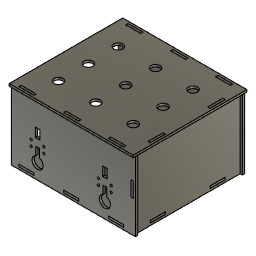
Chasis 4 with motor slots (Autodesk Fusion 360 design; units mm, degrees)
Autodesk Fusion 360 part; units mm, degrees
sketch "Sketch1" plane through (0, 0, 0) normal (0, 0, 1) x (1, 0, 0)
  line L0 (0, 0) -> (160, 0)
  line L1 (160, 0) -> (160, 140)
  line L2 (160, 140) -> (0, 140)
  line L3 (0, 140) -> (0, 0)
  line L4 (70, 0) -> (90, 0)
  line L5 (90, 0) -> (90, -3)
  line L6 (90, -3) -> (70, -3)
  line L7 (70, -3) -> (70, 0)
  line L8 (80, 0) -> (80, 24.5261)
  line L9 (0, 70) -> (20, 70)
  line L10 (150, -3) -> (130, -3)
  line L11 (130, -3) -> (130, 0)
  line L12 (150, 0) -> (150, -3)
  line L13 (30, -3) -> (10, -3)
  line L14 (10, -3) -> (10, 0)
  line L15 (30, 0) -> (30, -3)
  line L16 (0, 50) -> (0, 70)
  line L17 (10, 143) -> (10, 140)
  line L18 (30, 143) -> (10, 143)
  line L19 (30, 140) -> (30, 143)
  line L20 (70, 143) -> (70, 140)
  line L21 (90, 143) -> (70, 143)
  line L22 (90, 140) -> (90, 143)
  line L23 (130, 143) -> (130, 140)
  line L24 (150, 143) -> (130, 143)
  line L25 (150, 140) -> (150, 143)
  line L26 (160, 120) -> (163, 120)
  line L27 (163, 120) -> (163, 100)
  line L28 (163, 100) -> (160, 100)
  line L29 (160, 40) -> (163, 40)
  line L30 (163, 40) -> (163, 20)
  line L31 (163, 20) -> (160, 20)
  dimension "d1" = 140
  dimension "d2" = 3
  dimension "d3" = 20
  dimension "d6" = 0
  dimension "d7" = 60
  dimension "d71" = 140
  dimension "d72" = 140
  constraint horizontal L0
  constraint vertical L1
  constraint horizontal L2
  constraint vertical L3
  constraint coincident L0.start L3.end
  constraint horizontal L4
  constraint vertical L5
  constraint horizontal L6
  constraint vertical L7
  constraint coincident L0 L4.start
  constraint midpoint L0 L8.start
  constraint perpendicular L4 L8
  constraint midpoint L3 L9.start
  constraint perpendicular L3 L9
  constraint vertical L16
  constraint coincident L3 L9.start
  constraint symmetric L4.start L9 L20.end
  constraint symmetric L4.end L9 L22.start
  constraint symmetric L5.end L9 L21.start
  constraint symmetric L6.end L9 L20.start
  constraint symmetric L9 L10.start L24.start
  constraint symmetric L9 L10.end L23.start
  constraint symmetric L9 L11.end L23.end
  constraint symmetric L9 L12.start L25.start
  constraint symmetric L9 L13.start L18.start
  constraint symmetric L9 L13.end L17.start
  constraint symmetric L9 L14.end L17.end
  constraint symmetric L9 L15.start L19.start
  measures "d1" distance of L0.end L1.end
  measures "d2" distance of L4.end L5.end
  measures "d3" distance of L5.end L6.end
  measures "d71" distance of L0.end L1.end
  measures "d72" distance of L0.end L1.end
extrude "Extrude1" add sketch "Sketch1" along normal blind 3 makes body 1
sketch "Sketch2" plane through (0, 0, 0) normal (0, -1, 0) x (1, 0, 0)
  line L0 (0, 0) -> (10, 0)
  line L1 (10, 0) -> (10, 3)
  line L2 (10, 3) -> (0, 3)
  line L3 (0, 3) -> (0, 0)
  line L4 (0, -5) -> (168, -5)
  line L5 (168, -5) -> (168, 90)
  line L6 (168, 90) -> (0, 90)
  line L7 (0, 90) -> (0, -5)
  line L8 (70, 90) -> (90, 90)
  line L9 (90, 90) -> (90, 93)
  line L10 (90, 93) -> (70, 93)
  line L11 (70, 93) -> (70, 90)
  line L12 (30, 93) -> (10, 93)
  line L13 (10, 93) -> (10, 90)
  line L14 (30, 90) -> (30, 93)
  line L15 (150, 93) -> (130, 93)
  line L16 (130, 93) -> (130, 90)
  line L17 (150, 90) -> (150, 93)
  line L18 (0, -5) -> (168, -5)
  line L19 (168, -5) -> (168, -3)
  line L20 (168, -3) -> (0, -3)
  line L21 (0, -3) -> (0, -5)
  dimension "d15" = 168
  dimension "d16" = 95
  dimension "d17" = 20
  dimension "d18" = 3
  dimension "d21" = 60
  dimension "d22" = 0
  dimension "d85" = 2
  constraint horizontal L4
  constraint vertical L5
  constraint horizontal L6
  constraint vertical L7
  constraint horizontal L8
  constraint vertical L9
  constraint horizontal L10
  constraint vertical L11
  constraint coincident L6 L8.start
  constraint horizontal L18
  constraint vertical L19
  constraint horizontal L20
  constraint vertical L21
  measures "d15" distance of L4.start L4.end
  measures "d16" distance of L4.end L5.end
  measures "d17" distance of L9.end L10.end
  measures "d18" distance of L8.end L9.end
  measures "d85" distance of L4.start L20.end
extrude "Extrude2" add sketch "Sketch2" along normal blind 3 separate body makes body 2
sketch "Sketch3" plane through (160, 0, 0) normal (1, 0, 0) x (0, 1, 0)
  line L0 (0, 0) -> (20, 0)
  line L1 (20, 0) -> (20, 3)
  line L2 (20, 3) -> (0, 3)
  line L3 (0, 3) -> (0, 0)
  line L4 (0, -5) -> (140, -5)
  line L5 (140, -5) -> (140, 90)
  line L6 (140, 90) -> (0, 90)
  line L7 (0, 90) -> (0, -5)
  line L8 (20, 90) -> (40, 90)
  line L9 (40, 90) -> (40, 93)
  line L10 (40, 93) -> (20, 93)
  line L11 (20, 93) -> (20, 90)
  line L12 (100, 90) -> (120, 90)
  line L13 (120, 90) -> (120, 93)
  line L14 (120, 93) -> (100, 93)
  line L15 (100, 93) -> (100, 90)
  line L16 (0, 40) -> (-3, 40)
  line L17 (-3, 40) -> (-3, 60)
  line L18 (-3, 60) -> (0, 60)
  line L19 (0, 60) -> (0, 40)
  line L20 (140, 40) -> (143, 40)
  line L21 (143, 40) -> (143, 60)
  line L22 (143, 60) -> (140, 60)
  line L23 (140, 60) -> (140, 40)
  dimension "d33" = 20
  dimension "d34" = 3
  dimension "d35" = 3
  dimension "d36" = 3
  dimension "d37" = 20
  dimension "d38" = 3
  dimension "d74" = 140
  constraint horizontal L4
  constraint vertical L5
  constraint horizontal L6
  constraint vertical L7
  constraint horizontal L8
  constraint vertical L9
  constraint horizontal L10
  constraint vertical L11
  constraint coincident L6 L8.start
  constraint horizontal L12
  constraint vertical L13
  constraint horizontal L14
  constraint vertical L15
  constraint coincident L6 L12.start
  constraint horizontal L16
  constraint vertical L17
  constraint horizontal L18
  constraint vertical L19
  constraint coincident L7 L16.start
  constraint horizontal L20
  constraint vertical L21
  constraint horizontal L22
  constraint vertical L23
  constraint coincident L5 L20.start
  measures "d33" distance of L8.start L8.end
  measures "d34" distance of L8.start L10.end
  measures "d35" distance of L12.start L14.end
  measures "d36" distance of L16.start L16.end
  measures "d37" distance of L16.start L18.end
  measures "d38" distance of L20.start L20.end
  measures "d74" distance of L5 L7
extrude "Extrude5" add sketch "Sketch3" along normal blind 3 separate body contours L5 L20 L21 L22 L23 makes body 3
extrude "Extrude3" add sketch "Sketch3" along normal blind 3 separate body contours L0 L1 L2 L3 L7 | L0 L1 L2 L4 L5 L6 L7 L8 L12 L19 L23 | L7 L16 L17 L18 L19 | L6 L8 L9 L10 L11 | L6 L12 L13 L14 L15 makes body 4
sketch "Sketch5" plane through (0, 140, 0) normal (0, 1, 0) x (-1, 0, 0)
  line L0 (-160, 0) -> (-150, 0)
  line L1 (-150, 0) -> (-150, 3)
  line L2 (-150, 3) -> (-160, 3)
  line L3 (-160, 3) -> (-160, 0)
  line L4 (-168, -5) -> (0, -5)
  line L5 (0, -5) -> (0, 90)
  line L6 (0, 90) -> (-168, 90)
  line L7 (-168, 90) -> (-168, -5)
  line L8 (-150, 90) -> (-130, 90)
  line L9 (-130, 90) -> (-130, 93)
  line L10 (-130, 93) -> (-150, 93)
  line L11 (-150, 93) -> (-150, 90)
  line L12 (-90, 90) -> (-70, 90)
  line L13 (-70, 90) -> (-70, 78)
  line L14 (-70, 78) -> (-90, 78)
  line L15 (-90, 78) -> (-90, 90)
  line L16 (-30, 90) -> (-10, 90)
  line L17 (-10, 90) -> (-10, 78)
  line L18 (-10, 78) -> (-30, 78)
  line L19 (-30, 78) -> (-30, 90)
  dimension "d41" = 20
  dimension "d42" = 3
  constraint horizontal L4
  constraint vertical L5
  constraint horizontal L6
  constraint vertical L7
  constraint horizontal L8
  constraint vertical L9
  constraint horizontal L10
  constraint vertical L11
  constraint coincident L6 L8.start
  constraint horizontal L12
  constraint vertical L13
  constraint horizontal L14
  constraint vertical L15
  constraint coincident L6 L12.start
  constraint horizontal L16
  constraint vertical L17
  constraint horizontal L18
  constraint vertical L19
  constraint coincident L6 L16.start
  measures "d41" distance of L8.start L8.end
  measures "d42" distance of L8.start L10.end
combine "Combine1" operation add target body 4 tool bodies 3
combine "Combine2" [no effect]
sketch "Sketch7" plane through (0, 0, 90) normal (0, 0, 1) x (-1, 0, 0)
  line L0 (-10, 0) -> (0, 0)
  line L1 (0, 0) -> (0, 3)
  line L2 (0, 3) -> (-10, 3)
  line L3 (-10, 3) -> (-10, 0)
  line L4 (0, -128) -> (-168, -128)
  line L5 (-168, -128) -> (-168, 28)
  line L6 (-168, 28) -> (0, 28)
  line L7 (0, 28) -> (0, -128)
  dimension "d73" = 156
  constraint horizontal L4
  constraint vertical L5
  constraint horizontal L6
  constraint vertical L7
  measures "d73" distance of L4.start L6.end
extrude "Extrude8" add sketch "Sketch7" along normal blind 3 separate body makes body 5
combine "Combine4" operation cut target body 2 tool bodies 1 keep tools
combine "Combine5" operation cut target body 4 tool bodies 1 keep tools
combine "Combine6" operation cut target body 5 tool bodies 1 keep tools
combine "Combine7" operation cut target body 5 tool bodies 2 keep tools
combine "Combine8" operation cut target body 5 tool bodies 4 keep tools
combine "Combine9" operation cut target body 2 tool bodies 4 keep tools
sketch "Sketch8" plane through (0, -3, 0) normal (0, -1, 0) x (1, 0, 0)
  line L0 (160, 40) -> (160, 60)
  line L1 (160, 60) -> (163, 60)
  line L2 (163, 60) -> (163, 40)
  line L3 (163, 40) -> (160, 40)
  line L4 (130, 0) -> (130, 3)
  line L5 (130, 3) -> (150, 3)
  line L6 (150, 3) -> (150, 0)
  line L7 (150, 0) -> (130, 0)
  line L8 (70, 0) -> (70, 3)
  line L9 (70, 3) -> (90, 3)
  line L10 (90, 3) -> (90, 0)
  line L11 (90, 0) -> (70, 0)
  line L12 (10, 0) -> (10, 3)
  line L13 (10, 3) -> (30, 3)
  line L14 (30, 3) -> (30, 0)
  line L15 (30, 0) -> (10, 0)
  line L16 (150, 90) -> (150, 93)
  line L17 (150, 93) -> (130, 93)
  line L18 (130, 93) -> (130, 90)
  line L19 (130, 90) -> (90, 90)
  line L20 (90, 90) -> (90, 93)
  line L21 (90, 93) -> (70, 93)
  line L22 (70, 93) -> (70, 90)
  line L23 (70, 90) -> (30, 90)
  line L24 (30, 90) -> (30, 93)
  line L25 (30, 93) -> (10, 93)
  line L26 (10, 93) -> (10, 90)
  line L27 (10, 90) -> (0, 90)
  line L28 (0, 90) -> (0, -5)
  line L29 (0, -5) -> (168, -5)
  line L30 (168, -5) -> (168, 90)
  line L31 (168, 90) -> (150, 90)
  circle A0 centre (35, 17) radius 7.5
  circle A1 centre (125, 17) radius 7.5
  dimension "d54" = 15
  dimension "d55" = 15
  measures "d54" diameter of A1
  measures "d55" diameter of A0
sketch "Sketch9" plane through (0, 0, 93) normal (0, 0, 1) x (-1, 0, 0)
  line L0 (-10, 0) -> (-30, 0)
  line L1 (-30, 0) -> (-30, 3)
  line L2 (-30, 3) -> (-10, 3)
  line L3 (-10, 3) -> (-10, 0)
  line L4 (-70, 0) -> (-90, 0)
  line L5 (-90, 0) -> (-90, 3)
  line L6 (-90, 3) -> (-70, 3)
  line L7 (-70, 3) -> (-70, 0)
  line L8 (-130, 0) -> (-150, 0)
  line L9 (-150, 0) -> (-150, 3)
  line L10 (-150, 3) -> (-130, 3)
  line L11 (-130, 3) -> (-130, 0)
  line L12 (0, 28) -> (-168, 28)
  line L13 (-168, 28) -> (-168, -128)
  line L14 (-168, -128) -> (0, -128)
  line L15 (0, -128) -> (0, 28)
  circle A0 centre (-30, -90) radius 6
  circle A1 centre (-80, -90) radius 6
  circle A2 centre (-130, -90) radius 6
  circle A3 centre (-30, -50) radius 6
  circle A4 centre (-80, -50) radius 6
  circle A5 centre (-130, -50) radius 6
  circle A6 centre (-30, -10) radius 6
  circle A7 centre (-80, -10) radius 6
  circle A8 centre (-130, -10) radius 6
  line L16 (-160, -20) -> (-160, -40)
  line L17 (-160, -40) -> (-163, -40)
  line L18 (-163, -40) -> (-163, -20)
  line L19 (-163, -20) -> (-160, -20)
  line L20 (-160, -100) -> (-160, -120)
  line L21 (-160, -120) -> (-163, -120)
  line L22 (-163, -120) -> (-163, -100)
  line L23 (-163, -100) -> (-160, -100)
  dimension "d58" = 12
  dimension "d61" = -100
  dimension "d62" = 0
  dimension "d65" = 0
  dimension "d66" = 80
  measures "d58" diameter of A0
extrude "Extrude10" cut sketch "Sketch9" against normal blind 3 contours A0 | A1 | A2 | A3 | A4 | A5 | A6 | A7 | A8 bodies 5
extrude "Extrude11" cut sketch "Sketch9" against normal blind 86 contours A1 | A5 | A7 bodies 1
copy_body "CopyPasteBodies1" bodies 2 makes body 6
move_body "Move1" bodies 6 to x (1, 0, 0) y (0, 1, 0) z (0, 0, 1) at (0, 120, 0)
move_body "Move2" bodies 6 to x (1, 0, 0) y (0, 1, 0) z (0, 0, 1) at (0, 3, 0)
move_body "Move3" bodies 5 to x (1, 0, 0) y (0, 1, 0) z (0, 0, 1) at (0, 0, 10)
move_body "Move4" bodies 6 to x (1, 0, 0) y (0, 1, 0) z (0, 0, 1) at (0, 10, 0)
move_body "Move5" bodies 2 to x (1, 0, 0) y (0, 1, 0) z (0, 0, 1) at (0, -10, 0)
move_body "Move6" bodies 4 to x (1, 0, 0) y (0, 1, 0) z (0, 0, 1) at (10, 0, 0)
move_body "Move7" bodies 6 to x (1, 0, 0) y (0, 1, 0) z (0, 0, 1) at (0, 10, 0)
move_body "Move8" bodies 2 to x (1, 0, 0) y (0, 1, 0) z (0, 0, 1) at (0, 10, 0)
move_body "Move9" bodies 5 to x (1, 0, 0) y (0, 1, 0) z (0, 0, 1) at (0, 20, -10)
move_body "Move10" bodies 5 to x (1, 0, 0) y (0, 1, 0) z (0, 0, 1) at (0, 0, 10)
extrude "Extrude12" add 1 faces at (10, 19, 102) along direction (1, 0, 0) blind 20 on bodies 5 bodies 5
extrude "Extrude13" add 1 faces at (70, 19, 102) along direction (1, 0, 0) blind 20 on bodies 5 bodies 5
extrude "Extrude14" add 1 faces at (130, 19, 102) along direction (1, 0, 0) blind 20 on bodies 5 bodies 5
extrude "Extrude15" add 1 faces at (161, 140, 101) along direction (0, -1, 0) blind 20 on bodies 5 bodies 5
extrude "Extrude16" add 1 faces at (161, 60, 101) along direction (0, -1, 0) blind 20 on bodies 5 bodies 5
move_body "Move11" bodies 4 to x (1, 0, 0) y (0, 1, 0) z (0, 0, 1) at (-10, 0, 0)
move_body "Move12" bodies 5 to x (1, 0, 0) y (0, 1, 0) z (0, 0, 1) at (0, 0, -10)
move_body "Move13" bodies 5 to x (1, 0, 0) y (0, 1, 0) z (0, 0, 1) at (0, 0, 10)
move_body "Move14" bodies 5 to x (1, 0, 0) y (0, 1, 0) z (0, 0, 1) at (0, 0, -10)
combine "Combine11" operation cut target body 5 tool bodies 6 keep tools
combine "Combine12" operation cut target body 5 tool bodies 4 keep tools
combine "Combine13" operation cut target body 5 tool bodies 2 keep tools
sketch "Sketch10" plane through (0, -3, 0) normal (0, -1, 0) x (1, 0, 0)
  line L0 (160, 40) -> (160, 60)
  line L1 (160, 60) -> (163, 60)
  line L2 (163, 60) -> (163, 40)
  line L3 (163, 40) -> (160, 40)
  line L4 (130, 0) -> (130, 3)
  line L5 (130, 3) -> (150, 3)
  line L6 (150, 3) -> (150, 0)
  line L7 (150, 0) -> (130, 0)
  line L8 (70, 0) -> (70, 3)
  line L9 (70, 3) -> (90, 3)
  line L10 (90, 3) -> (90, 0)
  line L11 (90, 0) -> (70, 0)
  line L12 (10, 0) -> (10, 3)
  line L13 (10, 3) -> (30, 3)
  line L14 (30, 3) -> (30, 0)
  line L15 (30, 0) -> (10, 0)
  line L16 (150, 90) -> (150, 93)
  line L17 (150, 93) -> (130, 93)
  line L18 (130, 93) -> (130, 90)
  line L19 (130, 90) -> (90, 90)
  line L20 (90, 90) -> (90, 93)
  line L21 (90, 93) -> (70, 93)
  line L22 (70, 93) -> (70, 90)
  line L23 (70, 90) -> (30, 90)
  line L24 (30, 90) -> (30, 93)
  line L25 (30, 93) -> (10, 93)
  line L26 (10, 93) -> (10, 90)
  line L27 (10, 90) -> (0, 90)
  line L28 (0, 90) -> (0, -5)
  line L29 (0, -5) -> (168, -5)
  line L30 (168, -5) -> (168, 90)
  line L31 (168, 90) -> (150, 90)
  line L32 (0, -5) -> (168, -5)
  line L33 (168, -5) -> (168, -3)
  line L34 (168, -3) -> (0, -3)
  line L35 (0, -3) -> (0, -5)
  dimension "d86" = 2
  constraint horizontal L32
  constraint vertical L33
  constraint horizontal L34
  constraint vertical L35
  constraint coincident L28.end L29.start
  measures "d86" distance of L28.end L34.end
extrude "Extrude17" cut sketch "Sketch10" against normal blind 146 contours L28 L29 L30 L32 L33 L34 L35 bodies 2 4 6
sketch "Sketch11" plane through (0, -3, 0) normal (0, -1, 0) x (1, 0, 0)
  line L0 (0, -3) -> (168, -3)
  line L1 (168, -3) -> (168, 90)
  line L2 (168, 90) -> (150, 90)
  line L3 (150, 90) -> (150, 93)
  line L4 (150, 93) -> (130, 93)
  line L5 (130, 93) -> (130, 90)
  line L6 (130, 90) -> (90, 90)
  line L7 (90, 90) -> (90, 93)
  line L8 (90, 93) -> (70, 93)
  line L9 (70, 93) -> (70, 90)
  line L10 (70, 90) -> (30, 90)
  line L11 (30, 90) -> (30, 93)
  line L12 (30, 93) -> (10, 93)
  line L13 (10, 93) -> (10, 90)
  line L14 (10, 90) -> (0, 90)
  line L15 (0, 90) -> (0, -3)
  line L16 (160, 40) -> (160, 60)
  line L17 (160, 60) -> (163, 60)
  line L18 (163, 60) -> (163, 40)
  line L19 (163, 40) -> (160, 40)
  line L20 (130, 0) -> (130, 3)
  line L21 (130, 3) -> (150, 3)
  line L22 (150, 3) -> (150, 0)
  line L23 (150, 0) -> (130, 0)
  line L24 (70, 0) -> (70, 3)
  line L25 (70, 3) -> (90, 3)
  line L26 (90, 3) -> (90, 0)
  line L27 (90, 0) -> (70, 0)
  line L28 (10, 0) -> (10, 3)
  line L29 (10, 3) -> (30, 3)
  line L30 (30, 3) -> (30, 0)
  line L31 (30, 0) -> (10, 0)
  line L32 (168, -3) -> (166, -3)
  line L33 (166, -3) -> (166, 93)
  line L34 (166, 93) -> (168, 93)
  line L35 (168, 93) -> (168, -3)
  constraint horizontal L32
  constraint vertical L33
  constraint horizontal L34
  constraint vertical L35
  constraint coincident L0.end L1.start
extrude "Extrude18" cut sketch "Sketch11" against normal blind 146 contours L0 L1 L2 L32 L33 L35 | L2 L33 L34 L35 bodies 2 5 6
sketch "Sketch12" plane through (0, 0, 93) normal (0, 0, 1) x (-1, 0, 0)
  line L0 (-168, 3) -> (-166, 3)
  line L1 (-166, 3) -> (-166, -143)
  line L2 (-166, -143) -> (-168, -143)
  line L3 (-168, -143) -> (-168, -148)
  line L4 (-168, -148) -> (0, -148)
  line L5 (0, -148) -> (0, 8)
  line L6 (0, 8) -> (-168, 8)
  line L7 (-168, 8) -> (-168, 3)
  circle A0 centre (-130, -30) radius 6
  circle A1 centre (-80, -70) radius 6
  circle A2 centre (-30, -110) radius 6
  circle A3 centre (-30, -70) radius 6
  circle A4 centre (-80, -30) radius 6
  circle A5 centre (-130, -70) radius 6
  circle A6 centre (-80, -110) radius 6
  circle A7 centre (-130, -110) radius 6
  circle A8 centre (-30, -30) radius 6
  line L8 (-130, -143) -> (-150, -143)
  line L9 (-150, -143) -> (-150, -140)
  line L10 (-150, -140) -> (-130, -140)
  line L11 (-130, -140) -> (-130, -143)
  line L12 (-70, -143) -> (-90, -143)
  line L13 (-90, -143) -> (-90, -140)
  line L14 (-90, -140) -> (-70, -140)
  line L15 (-70, -140) -> (-70, -143)
  line L16 (-10, -143) -> (-30, -143)
  line L17 (-30, -143) -> (-30, -140)
  line L18 (-30, -140) -> (-10, -140)
  line L19 (-10, -140) -> (-10, -143)
  line L20 (-160, -100) -> (-160, -120)
  line L21 (-160, -120) -> (-163, -120)
  line L22 (-163, -120) -> (-163, -100)
  line L23 (-163, -100) -> (-160, -100)
  line L24 (-160, -20) -> (-160, -40)
  line L25 (-160, -40) -> (-163, -40)
  line L26 (-163, -40) -> (-163, -20)
  line L27 (-163, -20) -> (-160, -20)
  line L28 (-130, 0) -> (-150, 0)
  line L29 (-150, 0) -> (-150, 3)
  line L30 (-150, 3) -> (-130, 3)
  line L31 (-130, 3) -> (-130, 0)
  line L32 (-70, 0) -> (-90, 0)
  line L33 (-90, 0) -> (-90, 3)
  line L34 (-90, 3) -> (-70, 3)
  line L35 (-70, 3) -> (-70, 0)
  line L36 (-10, 0) -> (-30, 0)
  line L37 (-30, 0) -> (-30, 3)
  line L38 (-30, 3) -> (-10, 3)
  line L39 (-10, 3) -> (-10, 0)
  line L40 (-168, 3) -> (-166, 3)
  line L41 (-166, 3) -> (-166, 8)
  line L42 (-166, 8) -> (-168, 8)
  line L43 (-168, 8) -> (-168, 3)
  line L44 (-168, -148) -> (-166, -148)
  line L45 (-166, -148) -> (-166, -143)
  line L46 (-166, -143) -> (-168, -143)
  line L47 (-168, -143) -> (-168, -148)
  constraint horizontal L40
  constraint vertical L41
  constraint horizontal L42
  constraint vertical L43
  constraint coincident L6 L41.end
  constraint coincident L0.start L7.end
  constraint horizontal L44
  constraint vertical L45
  constraint horizontal L46
  constraint vertical L47
  constraint coincident L1.end L2.start
  constraint coincident L3.end L4.start
extrude "Extrude19" cut sketch "Sketch12" against normal blind 5 contours L0 L6 L7 L40 L41 L42 L43 | L2 L3 L4 L44 L45 L46 L47 bodies 5
sketch "Sketch13" plane through (0, 0, 93) normal (0, 0, 1) x (-1, 0, 0)
  line L0 (-166, 8) -> (-166, -148)
  line L1 (-166, -148) -> (0, -148)
  line L2 (0, -148) -> (0, 8)
  line L3 (0, 8) -> (-166, 8)
  circle A0 centre (-130, -30) radius 6
  circle A1 centre (-80, -70) radius 6
  circle A2 centre (-30, -110) radius 6
  circle A3 centre (-30, -70) radius 6
  circle A4 centre (-80, -30) radius 6
  circle A5 centre (-130, -70) radius 6
  circle A6 centre (-80, -110) radius 6
  circle A7 centre (-130, -110) radius 6
  circle A8 centre (-30, -30) radius 6
  line L4 (-130, -143) -> (-150, -143)
  line L5 (-150, -143) -> (-150, -140)
  line L6 (-150, -140) -> (-130, -140)
  line L7 (-130, -140) -> (-130, -143)
  line L8 (-70, -143) -> (-90, -143)
  line L9 (-90, -143) -> (-90, -140)
  line L10 (-90, -140) -> (-70, -140)
  line L11 (-70, -140) -> (-70, -143)
  line L12 (-10, -143) -> (-30, -143)
  line L13 (-30, -143) -> (-30, -140)
  line L14 (-30, -140) -> (-10, -140)
  line L15 (-10, -140) -> (-10, -143)
  line L16 (-160, -100) -> (-160, -120)
  line L17 (-160, -120) -> (-163, -120)
  line L18 (-163, -120) -> (-163, -100)
  line L19 (-163, -100) -> (-160, -100)
  line L20 (-160, -20) -> (-160, -40)
  line L21 (-160, -40) -> (-163, -40)
  line L22 (-163, -40) -> (-163, -20)
  line L23 (-163, -20) -> (-160, -20)
  line L24 (-130, 0) -> (-150, 0)
  line L25 (-150, 0) -> (-150, 3)
  line L26 (-150, 3) -> (-130, 3)
  line L27 (-130, 3) -> (-130, 0)
  line L28 (-70, 0) -> (-90, 0)
  line L29 (-90, 0) -> (-90, 3)
  line L30 (-90, 3) -> (-70, 3)
  line L31 (-70, 3) -> (-70, 0)
  line L32 (-10, 0) -> (-30, 0)
  line L33 (-30, 0) -> (-30, 3)
  line L34 (-30, 3) -> (-10, 3)
  line L35 (-10, 3) -> (-10, 0)
  line L36 (-166, -148) -> (0, -148)
  line L37 (0, -148) -> (0, -146)
  line L38 (0, -146) -> (-166, -146)
  line L39 (-166, -146) -> (-166, -148)
  line L40 (0, 8) -> (-166, 8)
  line L41 (-166, 8) -> (-166, 6)
  line L42 (-166, 6) -> (0, 6)
  line L43 (0, 6) -> (0, 8)
  dimension "d93" = 2
  dimension "d94" = 2
  constraint horizontal L36
  constraint vertical L37
  constraint horizontal L38
  constraint vertical L39
  constraint coincident L0.end L1.start
  constraint horizontal L40
  constraint vertical L41
  constraint horizontal L42
  constraint vertical L43
  constraint coincident L2.end L3.start
  measures "d93" distance of L0.end L38.end
  measures "d94" distance of L2.end L42.end
extrude "Extrude20" cut sketch "Sketch13" against normal blind 5 contours L0 L2 L3 L40 L41 L42 L43 | L0 L1 L2 L36 L37 L38 L39 bodies 5
extrude "Extrude21" cut sketch "Sketch8" against normal blind 146 contours A0 | A1 bodies 2 6
sketch "Sketch14" plane through (0, -3, 0) normal (0, -1, 0) x (1, 0, 0)
  circle A0 centre (35, 17) radius 7.5
  circle A1 centre (125, 17) radius 7.5
  line L0 (166, -3) -> (166, 90)
  line L1 (166, 90) -> (150, 90)
  line L2 (150, 90) -> (150, 93)
  line L3 (150, 93) -> (130, 93)
  line L4 (130, 93) -> (130, 90)
  line L5 (130, 90) -> (90, 90)
  line L6 (90, 90) -> (90, 93)
  line L7 (90, 93) -> (70, 93)
  line L8 (70, 93) -> (70, 90)
  line L9 (70, 90) -> (30, 90)
  line L10 (30, 90) -> (30, 93)
  line L11 (30, 93) -> (10, 93)
  line L12 (10, 93) -> (10, 90)
  line L13 (10, 90) -> (0, 90)
  line L14 (0, 90) -> (0, -3)
  line L15 (0, -3) -> (166, -3)
  line L16 (160, 40) -> (160, 60)
  line L17 (160, 60) -> (163, 60)
  line L18 (163, 60) -> (163, 40)
  line L19 (163, 40) -> (160, 40)
  line L20 (130, 0) -> (130, 3)
  line L21 (130, 3) -> (150, 3)
  line L22 (150, 3) -> (150, 0)
  line L23 (150, 0) -> (130, 0)
  line L24 (70, 0) -> (70, 3)
  line L25 (70, 3) -> (90, 3)
  line L26 (90, 3) -> (90, 0)
  line L27 (90, 0) -> (70, 0)
  line L28 (10, 0) -> (10, 3)
  line L29 (10, 3) -> (30, 3)
  line L30 (30, 3) -> (30, 0)
  line L31 (30, 0) -> (10, 0)
  circle A2 centre (26.5, 32) radius 1.5
  circle A3 centre (26.5, 40) radius 1.5
  circle A4 centre (43.5, 40) radius 1.5
  circle A5 centre (43.5, 32) radius 1.5
  line L32 (35, 17) -> (35, 47.5006)
  line L33 (125, 17) -> (125, 47.5006)
  line L34 (83, -3) -> (83, 54.1393)
  circle A6 centre (116.5, 40) radius 1.5
  circle A7 centre (133.5, 40) radius 1.5
  circle A8 centre (133.5, 32) radius 1.5
  circle A9 centre (116.5, 32) radius 1.5
  line L35 (32.5, 24.0711) -> (37.5, 24.0711)
  line L36 (37.5, 24.0711) -> (37.5, 35)
  line L37 (37.5, 35) -> (32.5, 35)
  line L38 (32.5, 35) -> (32.5, 24.0711)
  line L39 (32, 55) -> (38, 55)
  line L40 (32, 56.9597) -> (38, 56.9597)
  line L41 (38, 56.9597) -> (38, 57.0304)
  line L42 (38, 57.0304) -> (32, 57.0304)
  line L43 (32, 57.0304) -> (32, 56.9597)
  line L44 (32, 45.0304) -> (38, 45.0304)
  line L45 (38, 45.0304) -> (38, 45)
  line L46 (38, 45) -> (32, 45)
  line L47 (32, 45) -> (32, 45.0304)
  line L48 (38, 56.9597) -> (32, 56.9597)
  line L49 (32, 56.9597) -> (32, 57.0304)
  line L50 (32, 57.0304) -> (38, 57.0304)
  line L51 (38, 57.0304) -> (38, 56.9597)
  line L52 (32, 56.9597) -> (38, 56.9597)
  line L53 (38, 56.9597) -> (38, 45)
  line L54 (38, 45) -> (32, 45)
  line L55 (32, 45) -> (32, 56.9597)
  line L56 (128, 56.9597) -> (128, 45)
  line L57 (128, 56.9597) -> (122, 56.9597)
  line L58 (122, 45) -> (122, 56.9597)
  line L59 (128, 45) -> (122, 45)
  line L60 (127.5, 35) -> (122.5, 35)
  line L61 (122.5, 35) -> (122.5, 24.0711)
  line L62 (122.5, 24.0711) -> (127.5, 24.0711)
  line L63 (127.5, 24.0711) -> (127.5, 35)
  dimension "d99" = 3
  dimension "d100" = 3
  dimension "d103" = 43
  dimension "d104" = 35
  dimension "d105" = 3
  dimension "d106" = 3
  dimension "d107" = 17
  dimension "d108" = 17
  dimension "d111" = 3
  dimension "d112" = 3
  dimension "d113" = 3
  dimension "d114" = 3
  dimension "d115" = 17
  dimension "d116" = 17
  dimension "d118" = 26.5
  dimension "d125" = 5
  dimension "d126" = 2.5
  dimension "d128" = 10.9289
  dimension "d130" = 6
  dimension "d131" = 3
  dimension "d132" = 20
  dimension "d133" = 12
  dimension "d134" = 20.9289
  dimension "d135" = 5
  dimension "d136" = 20.9289
  dimension "d140" = 8.5
  dimension "d141" = 8.5
  dimension "d142" = 8.5
  dimension "d143" = 8.5
  constraint coincident A0.centre L32.start
  constraint parallel L16 L32
  constraint coincident A1.centre L33.start
  constraint perpendicular L13 L33
  constraint midpoint L15 L34.start
  constraint perpendicular L27 L34
  constraint horizontal L35
  constraint vertical L36
  constraint horizontal L37
  constraint vertical L38
  constraint coincident A0 L35.start
  constraint horizontal L39
  constraint horizontal L40
  constraint vertical L41
  constraint horizontal L42
  constraint vertical L43
  constraint horizontal L44
  constraint vertical L45
  constraint horizontal L46
  constraint vertical L47
  constraint horizontal L48
  constraint vertical L49
  constraint horizontal L50
  constraint vertical L51
  constraint horizontal L52
  constraint vertical L53
  constraint horizontal L54
  constraint vertical L55
  constraint horizontal L62
  constraint vertical L63
  constraint horizontal L60
  constraint vertical L61
  constraint horizontal L57
  constraint vertical L56
  constraint horizontal L59
  constraint vertical L58
  measures "d99" diameter of A2
  measures "d100" diameter of A3
  measures "d103" distance of L15 A3.centre
  measures "d104" distance of L15 A2.centre
  measures "d105" diameter of A4
  measures "d106" diameter of A5
  measures "d107" distance of A3.centre A4.centre
  measures "d108" distance of A2.centre A5.centre
  measures "d111" diameter of A9
  measures "d112" diameter of A6
  measures "d113" diameter of A7
  measures "d114" diameter of A8
  measures "d115" distance of A6.centre A7.centre
  measures "d116" distance of A9.centre A8.centre
  measures "d118" distance of L14 A2.centre
  measures "d125" distance of L36.end L37.end
  measures "d126" distance of A0.centre L36
  measures "d128" distance of L35.start L37.end
  measures "d130" distance of L39.start L39.end
  measures "d131" horizontal distance of A0.centre L39.start
  measures "d132" distance of L37 L39
  measures "d133" distance of L42 L44
  measures "d134" distance of L35 L54
  measures "d135" distance of L60.start L60.end
  measures "d136" distance of L59 L62
  measures "d140" horizontal distance of A5.centre A0.centre
  measures "d141" horizontal distance of A1.centre A8.centre
  measures "d142" horizontal distance of A4.centre A0.centre
  measures "d143" horizontal distance of A1.centre A7.centre
extrude "Extrude23" cut sketch "Sketch14" against normal blind 146 contours A0 L32 L36 L37 | A0 L32 L37 L38 | A1 L33 L60 L63 | A1 L33 L60 L61 | L39 L44 L53 L55 | L39 L40 L48 L52 L53 L55 | L56 L57 L58 L59 bodies 2 6
extrude "Extrude22" cut sketch "Sketch14" against normal blind 146 contours A2 | A3 | A4 | A5 | A6 | A7 | A8 | A9 bodies 2 6
